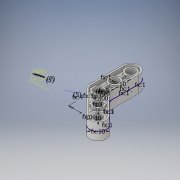
# Autodesk Inventor part: Bent beam 5-135
Saved by Autodesk Inventor 2019 (Build 230136000, 136)
## iProperties
Created: 2019-01-29
Part Number: Bent beam 5-135
Material: Generic
Document SubType Name: Modeling
Designer: Varga Daniel
Density: 1 g/cm^3
Appearance: Default
Author: Varga Daniel
Autodesk Inventor part; units mm, degrees
ref_plane "YZ Plane" through (0, 0, 0) normal (1, 0, 0) x (0, 1, 0)
ref_plane "XZ Plane" through (0, 0, 0) normal (0, 1, 0) x (-1, 0, 0)
ref_plane "XY Plane" through (0, 0, 0) normal (0, 0, 1) x (1, 0, 0)
derived "Base_part.ipt"
sketch "Sketch1" plane through (0, 0, 0) normal (0, 1, 0) x (-1, 0, 0)
  line L0 (5, 0) -> (25, 0)
  line L1 (30, 5) -> (30, 25)
  line L2 (25, 30) -> (5, 30)
  line L3 (0, 25) -> (0, 5)
  line L4 (5, 29) -> (25, 29)
  line L5 (29, 25) -> (29, 5)
  line L6 (25, 1) -> (5, 1)
  line L7 (1, 5) -> (1, 25)
  circle A0 centre (5, 5) radius 2.5
  circle A1 centre (5, 5) radius 3.5
  arc A2 (25, 0) -> (30, 5) centre (25, 5) ccw
  arc A3 (30, 25) -> (25, 30) centre (25, 25) ccw
  arc A4 (5, 30) -> (0, 25) centre (5, 25) ccw
  arc A5 (0, 5) -> (5, 0) centre (5, 5) ccw
  arc A6 (1, 5) -> (5, 1) centre (5, 5) ccw
  arc A7 (5, 29) -> (1, 25) centre (5, 25) ccw
  arc A8 (29, 25) -> (25, 29) centre (25, 25) ccw
  arc A9 (25, 1) -> (29, 5) centre (25, 5) ccw
  line L8 (49.1041, 15) -> (-27.081, 15) construction
  circle A10 centre (5, 15) radius 2.5
  circle A11 centre (5, 15) radius 3.5
  circle A12 centre (15, 5) radius 2.5
  circle A13 centre (15, 5) radius 3.5
  circle A14 centre (15, 15) radius 2.5
  circle A15 centre (15, 15) radius 3.5
  line L9 (1, 9.5) -> (1, 10.5)
  line L10 (29, 10.5) -> (29, 9.5)
  line L11 (31.1478, 10) -> (-2.4877, 10) construction
  line L12 (-2.8604, 5) -> (35.495, 5) construction
  line L13 (11.5359, 5.5) -> (8.4641, 5.5)
  line L14 (11.5359, 4.5) -> (8.4641, 4.5)
  line L15 (5, -2.5736) -> (5, 36.7522) construction
  line L16 (5.5, 8.4641) -> (5.5, 11.5359)
  line L17 (4.5, 8.4641) -> (4.5, 11.5359)
  line L18 (8.4641, 15.5) -> (11.5359, 15.5)
  line L19 (11.5359, 14.5) -> (8.4641, 14.5)
  line L20 (5.5, 1.5359) -> (5.5, 1)
  line L21 (4.5, 1.5359) -> (4.5, 1.0314)
  line L22 (1.5359, 4.5) -> (1.0314, 4.5)
  line L23 (1.5359, 5.5) -> (1, 5.5)
  line L24 (15, -1.4978) -> (15, 34.8784) construction
  line L25 (15.5, 8.4641) -> (15.5, 11.5359)
  line L26 (14.5, 11.5359) -> (14.5, 8.4641)
  line L27 (15.5, 1.5359) -> (15.5, 1)
  line L28 (14.5, 1.5359) -> (14.5, 1)
  line L29 (1.5359, 15.5) -> (1, 15.5)
  line L30 (1.5359, 14.5) -> (1, 14.5)
  line L31 (1, 10.5) -> (4.5, 10.5)
  line L32 (4.5, 10.5) -> (14.5, 10.5)
  line L33 (14.5, 9.5) -> (4.5, 9.5)
  line L34 (4.5, 9.5) -> (1, 9.5)
  line L35 (24.5, 8.4641) -> (24.5, 11.5359)
  line L36 (18.4641, 5.5) -> (21.5359, 5.5)
  line L37 (24.5, 10.5) -> (14.5, 10.5)
  line L38 (14.5, 9.5) -> (24.5, 9.5)
  circle A16 centre (25, 5) radius 2.5
  circle A17 centre (25, 5) radius 3.5
  line L39 (18.4641, 4.5) -> (21.5359, 4.5)
  line L40 (29, 9.5) -> (29, 10.5)
  line L41 (15.5, 11.5359) -> (15.5, 8.4641)
  line L42 (25.5, 8.4641) -> (25.5, 11.5359)
  line L43 (29, 10.5) -> (24.5, 10.5)
  line L44 (24.5, 9.5) -> (29, 9.5)
  line L45 (28.4641, 4.5) -> (28.9686, 4.5)
  line L46 (28.4641, 5.5) -> (29, 5.5)
  line L47 (15.5, 1.5359) -> (15.5, 1)
  line L48 (14.5, 1.5359) -> (14.5, 1)
  line L49 (24.5, 1.5359) -> (24.5, 1)
  line L50 (25.5, 1.5359) -> (25.5, 1.0314)
  line L51 (18.4641, 14.5) -> (21.5359, 14.5)
  line L52 (21.5359, 15.5) -> (18.4641, 15.5)
  circle A18 centre (25, 15) radius 2.5
  circle A19 centre (25, 15) radius 3.5
  line L53 (28.4641, 15.5) -> (29, 15.5)
  line L54 (28.4641, 14.5) -> (29, 14.5)
  line L55 (31.1478, 20) -> (-2.4877, 20) construction
  circle A20 centre (5, 25) radius 2.5
  circle A21 centre (5, 25) radius 3.5
  line L56 (15.5, 21.5359) -> (15.5, 18.4641)
  line L57 (15.5, 18.4641) -> (15.5, 21.5359)
  line L58 (14.5, 18.4641) -> (14.5, 21.5359)
  line L59 (24.5, 19.5) -> (14.5, 19.5)
  line L60 (15.5, 20.5) -> (25.5, 20.5)
  circle A22 centre (15, 25) radius 2.5
  circle A23 centre (15, 25) radius 3.5
  line L61 (11.5359, 25.5) -> (8.4641, 25.5)
  line L62 (11.5359, 24.5) -> (8.4641, 24.5)
  line L63 (4.5, 19.5) -> (14.5, 19.5)
  line L64 (15.5, 20.5) -> (5.5, 20.5)
  line L65 (18.4641, 24.5) -> (21.5359, 24.5)
  line L66 (18.4641, 25.5) -> (21.5359, 25.5)
  line L67 (15.5, 28.4641) -> (15.5, 29)
  line L68 (15.5, 28.4641) -> (15.5, 29)
  line L69 (14.5, 28.4641) -> (14.5, 29)
  line L70 (14.5, 28.4641) -> (14.5, 29)
  line L71 (1, 20.5) -> (1, 19.5)
  line L72 (5.5, 21.5359) -> (5.5, 18.4641)
  line L73 (4.5, 21.5359) -> (4.5, 18.4641)
  line L74 (1, 19.5) -> (4.5, 19.5)
  line L75 (5.5, 20.5) -> (1, 20.5)
  line L76 (5.5, 28.4641) -> (5.5, 29)
  line L77 (4.5, 28.4641) -> (4.5, 28.9686)
  line L78 (1.5359, 25.5) -> (1.0314, 25.5)
  line L79 (1.5359, 24.5) -> (1, 24.5)
  line L80 (24.5, 21.5359) -> (24.5, 18.4641)
  line L81 (29, 19.5) -> (29, 20.5)
  circle A24 centre (25, 25) radius 2.5
  circle A25 centre (25, 25) radius 3.5
  line L82 (24.5, 28.4641) -> (24.5, 29)
  line L83 (25.5, 28.4641) -> (25.5, 28.9686)
  line L84 (28.4641, 25.5) -> (28.9686, 25.5)
  line L85 (25.5, 21.5359) -> (25.5, 18.4641)
  line L86 (28.4641, 24.5) -> (29, 24.5)
  line L87 (25.5, 20.5) -> (29, 20.5)
  line L88 (29, 19.5) -> (24.5, 19.5)
  line L89 (29, 20.5) -> (29, 19.5)
  point P0 (0, 0)
  point P1 (30, 30)
  point P2 (0, 30)
  point P3 (5, 15)
  point P4 (5, 15)
  point P5 (15, 5)
  point P6 (15, 15)
  point P7 (5.5, 10.5)
  point P8 (5.5, 9.5)
  point P9 (14.5, 11.5359)
  point P10 (15.5, 10.5)
  point P11 (15.5, 9.5)
  point P12 (25, 5)
  point P13 (25, 5)
  point P14 (30, 0)
  point P15 (25.5, 9.5)
  point P16 (25.5, 10.5)
  point P17 (25, 15)
  point P18 (25, 15)
  point P19 (15, 25)
  point P20 (-2.8604, 25)
  point P21 (25, 25)
  point P22 (5, 25)
  point P23 (5, 25)
  point P24 (25, 25)
  point P25 (15.5, 19.5)
  point P26 (14.5, 18.4641)
  point P27 (24.5, 20.5)
  point P28 (15, 31.4978)
  point P29 (5, 32.5736)
  point P30 (5.5, 19.5)
  point P31 (14.5, 20.5)
  point P32 (4.5, 20.5)
  point P33 (25, 25)
  point P34 (25, 25)
  point P35 (25.5, 19.5)
sketch "Sketch2" plane through (0, 0, 0) normal (0, 1, 0) x (-1, 0, 0)
  circle A0 centre (25, 5) radius 3.5 construction
  circle A1 centre (25, 5) radius 2.5 construction
  line L0 (24.5, 8.4641) -> (24.5, 11.5359) construction
  line L1 (25.5, 8.4641) -> (25.5, 11.5359) construction
  arc A2 (25, 1) -> (29, 5) centre (25, 5) ccw construction
  arc A3 (25, 0) -> (30, 5) centre (25, 5) ccw construction
  line L2 (24.5, 10.5) -> (14.5, 10.5) construction
  line L3 (14.5, 9.5) -> (24.5, 9.5) construction
  line L4 (-9.8186, -3.1319) -> (-9.8186, -21.0609)
  line L5 (0.1814, -1.0609) -> (0.1814, -21.0609)
  line L6 (0.1814, -21.0609) -> (-9.8186, -21.0609) construction
  line L7 (-0.8186, -1.0609) -> (-0.8186, -21.0609)
  line L8 (-8.8186, -3.1319) -> (-8.8186, -21.0609)
  line L9 (-4.8186, -1.0609) -> (-4.8186, -21.0609) construction
  line L10 (-9.8186, -3.1319) -> (-22.4963, 9.5457)
  line L11 (-21.7892, 10.2528) -> (-9.1115, -2.4248)
  line L12 (-4.8186, -1.0609) -> (-2.3335, -3.5461) construction
  line L13 (-9.8186, -3.1319) -> (9.7269, 4.9641) construction
  arc A4 (-8.8186, -3.1319) -> (-9.1115, -2.4248) centre (-9.8186, -3.1319) ccw
  arc A5 (0.1814, -1.0609) -> (-1.2831, 2.4747) centre (-4.8186, -1.0609) ccw
  line L14 (-1.2831, 2.4747) -> (-15.4252, 16.6168)
  line L15 (-1.9902, 1.7675) -> (-16.1324, 15.9097)
  arc A6 (-0.8186, -1.0609) -> (-1.9902, 1.7675) centre (-4.8186, -1.0609) ccw
  line L16 (-15.4252, 16.6168) -> (-22.4963, 9.5457) construction
  circle A7 centre (-4.8186, -1.0609) radius 2.5
  circle A8 centre (-4.8186, -1.0609) radius 3.5
  arc A9 (-9.8186, -21.0609) -> (0.1814, -21.0609) centre (-4.8186, -21.0609) ccw
  arc A10 (-8.8186, -21.0609) -> (-0.8186, -21.0609) centre (-4.8186, -21.0609) ccw
  circle A11 centre (-11.8897, 6.0102) radius 2.5
  circle A12 centre (-11.8897, 6.0102) radius 3.5
  arc A13 (-15.4252, 16.6168) -> (-22.4963, 9.5457) centre (-18.9608, 13.0813) ccw
  arc A14 (-16.1324, 15.9097) -> (-21.7892, 10.2528) centre (-18.9608, 13.0813) ccw
  circle A15 centre (-18.9608, 13.0813) radius 2.5
  circle A16 centre (-18.9608, 13.0813) radius 3.5
  circle A17 centre (-4.8186, -11.0609) radius 2.5
  circle A18 centre (-4.8186, -11.0609) radius 3.5
  circle A19 centre (-4.8186, -21.0609) radius 2.5
  circle A20 centre (-4.8186, -21.0609) radius 3.5
  line L17 (-4.3186, -4.525) -> (-4.3186, -7.5968)
  line L18 (-5.3186, -7.5968) -> (-5.3186, -4.525)
  line L19 (-5.3186, -14.525) -> (-5.3186, -17.5968)
  line L20 (-4.3186, -14.525) -> (-4.3186, -17.5968)
  line L21 (-5.3186, -25.0295) -> (-5.3186, -24.525)
  line L22 (-4.3186, -25.0295) -> (-4.3186, -24.525)
  line L23 (-7.6217, 1.0351) -> (-9.7938, 3.2071)
  line L24 (-9.0867, 3.9143) -> (-6.9146, 1.7422)
  line L25 (-14.6928, 8.1061) -> (-16.8648, 10.2782)
  line L26 (-16.1577, 10.9853) -> (-13.9857, 8.8132)
  line L27 (-21.7638, 15.1772) -> (-22.1206, 15.5339)
  line L28 (-21.0567, 15.8843) -> (-21.4135, 16.2411)
  line L29 (-4.8186, -11.0609) -> (-8.8186, -11.0609) construction
  line L30 (-8.2827, -11.5609) -> (-8.8186, -11.5609)
  line L31 (-8.2827, -10.5609) -> (-8.8186, -10.5609)
  line L32 (-1.3545, -11.5609) -> (-0.8186, -11.5609)
  line L33 (-1.3545, -10.5609) -> (-0.8186, -10.5609)
  line L34 (-8.2827, -21.5609) -> (-8.7873, -21.5609)
  line L35 (-8.2827, -20.5609) -> (-8.8186, -20.5609)
  line L36 (-1.3545, -21.5609) -> (-0.85, -21.5609)
  line L37 (-0.8186, -20.5609) -> (-1.3545, -20.5609)
  line L38 (-11.8897, 6.0102) -> (-14.7181, 3.1818) construction
  line L39 (-14.3646, 2.8282) -> (-13.9857, 3.2071)
  line L40 (-14.6928, 3.9143) -> (-15.0717, 3.5353)
  line L41 (-9.0867, 8.1061) -> (-8.7077, 8.4851)
  line L42 (-9.7938, 8.8132) -> (-9.4148, 9.1922)
  line L43 (-21.4357, 9.8993) -> (-21.0567, 10.2782)
  line L44 (-21.7638, 10.9853) -> (-22.1206, 10.6286)
  line L45 (-16.1577, 15.1772) -> (-15.7788, 15.5561)
  line L46 (-16.8648, 15.8843) -> (-16.5081, 16.2411)
  line L47 (-0.9608, -0.0041) -> (-1.4269, -0.1972)
  line L48 (-1.3435, 0.9198) -> (-1.8096, 0.7267)
  point P0 (-5.3186, 2.4032)
  point P1 (-4.3186, 2.4032)
  point P2 (-2.7227, -3.8639)
  point P3 (-2.0156, -3.1568)
  dimension "d19" = 7
  dimension "d1" = 5
  dimension "d2" = 7
  dimension "d5" = 10
  dimension "d7" = 1
  dimension "d8" = 1
  dimension "d9" = 135
  dimension "d10" = 1
  dimension "d11" = 1
  dimension "d12" = 5
  dimension "d13" = 10
  dimension "d14" = 1
  dimension "d16" = 5
  dimension "d17" = 4
  dimension "d18" = 5
  dimension "d50" = 10
  dimension "d64" = 10
  dimension "d71" = 10
  dimension "d78" = 10
  dimension "d83" = 1
  dimension "d84" = 1
  dimension "d85" = 1
  dimension "d86" = 1
  dimension "d87" = 1
  dimension "d88" = 1
  dimension "d96" = 1
  constraints: 90 end point, 24 point on circle, 22 parallel, 19 point on line, 16 collinear, 12 centre point, 8 coincident, 8 tangent, 7 vertical, 4 perpendicular, 3 midpoint, 76 other
  measures "d1" diameter of A1
  measures "d2" diameter of A0
  measures "d5" distance between parallel lines of L4 L5
  measures "d7" distance between parallel lines of L5 L7
  measures "d8" distance between parallel lines of L4 L8
  measures "d9" angle of L9 L12
  measures "d10" distance between parallel lines of L10 L11
  measures "d11" radius of A4
  measures "d12" distance between parallel lines of L12 L10
  measures "d13" distance between parallel lines of L14 L10
  measures "d14" distance between parallel lines of L15 L14
  measures "d16" radius of A5
  measures "d17" radius of A6
  measures "d18" diameter of A7
  measures "d50" distance of A7.centre A11.centre
  measures "d64" distance of A11.centre A15.centre
  measures "d71" distance of A7.centre A17.centre
  measures "d78" distance of A17.centre A19.centre
  measures "d83" distance between parallel lines of L18 L17
  measures "d84" distance between parallel lines of L24 L23
  measures "d85" distance between parallel lines of L31 L30
  measures "d86" distance between parallel lines of L35 L34
  measures "d87" distance between parallel lines of L39 L40
  measures "d88" distance between parallel lines of L44 L43
  measures "d96" distance between parallel lines of L48 L47
extrude "Extrusion1" add sketch "Sketch2" along normal blind 5 contours L10 A13 L14 A5 L5 A9 L4
extrude "Extrusion2" add sketch "Sketch2" against normal blind 5 contours L10 A13 L14 A5 L5 A9 L4
extrude "Extrusion4" add sketch "Sketch2" along normal blind 4.2 contours L7 L32 A18 L33 | L47 A8 L48 A6 | A18 | A8 | L7 A10 L36 A20 L37 | A18 L18 A8 L17 | A20 | L20 A20 L19 A18 | L41 A12 L42 L15 | A8 L23 A12 L24 | A18 L30 L8 L31 | A12 | A10 L21 A20 L22 | L45 A16 L46 A14 L15 | A20 L34 A10 L8 L35 | A16 | A12 L25 A16 L26 | L39 L11 L40 A12 | L28 A16 L27 A14 | L43 L11 A14 L44 A16
extrude "Extrusion5" add sketch "Sketch2" against normal blind 4.2 contours L7 L32 A18 L33 | L47 A8 L48 A6 | A18 | A8 | L7 A10 L36 A20 L37 | A18 L18 A8 L17 | A20 | L20 A20 L19 A18 | L41 A12 L42 L15 | A8 L23 A12 L24 | A18 L30 L8 L31 | A12 | A10 L21 A20 L22 | L45 A16 L46 A14 L15 | A20 L34 A10 L8 L35 | A16 | A12 L25 A16 L26 | L39 L11 L40 A12 | L28 A16 L27 A14 | L43 L11 A14 L44 A16
extrude "Extrusion6" add sketch "Sketch2" along normal blind 2.7 contours L7 L33 A18 L17 A8 L47 A6 | L7 L37 A20 L20 A18 L32 | L48 A8 L24 A12 L41 L15 A6 | A18 L31 L8 A4 L11 L39 A12 L23 A8 L18 | A10 L22 A20 L36 | L19 A20 L35 L8 L30 A18 | L42 A12 L26 A16 L45 L15 | A10 L34 A20 L21 | L46 A16 L28 A14 | A12 L40 L11 L43 A16 L25 | L27 A16 L44 A14
extrude "Extrusion7" add sketch "Sketch2" against normal blind 2.7 contours L7 L33 A18 L17 A8 L47 A6 | L7 L37 A20 L20 A18 L32 | L48 A8 L24 A12 L41 L15 A6 | A18 L31 L8 A4 L11 L39 A12 L23 A8 L18 | A10 L22 A20 L36 | L19 A20 L35 L8 L30 A18 | L42 A12 L26 A16 L45 L15 | A10 L34 A20 L21 | L46 A16 L28 A14 | A12 L40 L11 L43 A16 L25 | L27 A16 L44 A14
equation "\"d19\" = d2"
equation "\"d7\" = Wall_thickness"
equation "\"d8\" = d7"
equation "\"d10\" = d7"
equation "\"d11\" = d7"
equation "\"d12\" = 0.5 * d5"
equation "\"d13\" = d5"
equation "\"d14\" = d7"
equation "\"d17\" = d16 - d7"
equation "\"d18\" = d1"
equation "\"d83\" = Inner_route_thickness"
equation "\"d84\" = Inner_route_thickness"
equation "\"d85\" = Inner_route_thickness"
equation "\"d86\" = Inner_route_thickness"
equation "\"d87\" = Inner_route_thickness"
equation "\"d88\" = Inner_route_thickness"
equation "\"d89\" = 0.5 * Overall_height"
equation "\"d91\" = 0.5 * Overall_height"
equation "\"Wall_thickness\" = 1"
equation "\"Inner_route_thickness\" = 1"
equation "\"Overall_height\" = 10"
body "Solid1"
